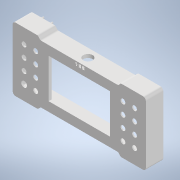
# Autodesk Inventor part: CONTROL_BOARD
Saved by Autodesk Inventor 2020 (Build 240168000, 168)
## iProperties
Created: 2020-06-05
Part Number: CONTROL_BOARD
Material: Generic
Document SubType Name: Modeling
Designer: Gebruiker
Density: 1 g/cm^3
Appearance: Default
Author: Gebruiker
Autodesk Inventor part; units mm, degrees
ref_plane "YZ Plane" through (0, 0, 0) normal (1, 0, 0) x (0, 1, 0)
ref_plane "XZ Plane" through (0, 0, 0) normal (0, 1, 0) x (-1, 0, 0)
ref_plane "XY Plane" through (0, 0, 0) normal (0, 0, 1) x (1, 0, 0)
sketch "Sketch1" plane through (0, 0, 0) normal (0, 0, 1) x (1, 0, 0)
  line L0 (-92.5, -50) -> (92.5, -50)
  line L1 (92.5, -50) -> (92.5, 50)
  line L2 (92.5, 50) -> (-92.5, 50)
  line L3 (-92.5, 50) -> (-92.5, -50)
  line L4 (-92.5, -50) -> (92.5, 50) construction
  line L5 (92.5, -50) -> (-92.5, 50) construction
  line L6 (70, 55) -> (115, 55)
  line L7 (115, 55) -> (115, 45)
  line L8 (115, 45) -> (70, 45)
  line L9 (70, 45) -> (70, 55)
  line L10 (70, 55) -> (115, 45) construction
  line L11 (115, 55) -> (70, 45) construction
  line L12 (70, -45) -> (115, -45)
  line L13 (115, -45) -> (115, -55)
  line L14 (115, -55) -> (70, -55)
  line L15 (70, -55) -> (70, -45)
  line L16 (70, -45) -> (115, -55) construction
  line L17 (115, -45) -> (70, -55) construction
  line L18 (-115, -45) -> (-70, -45)
  line L19 (-70, -45) -> (-70, -55)
  line L20 (-70, -55) -> (-115, -55)
  line L21 (-115, -55) -> (-115, -45)
  line L22 (-115, -45) -> (-70, -55) construction
  line L23 (-70, -45) -> (-115, -55) construction
  line L24 (-115, 55) -> (-70, 55)
  line L25 (-70, 55) -> (-70, 45)
  line L26 (-70, 45) -> (-115, 45)
  line L27 (-115, 45) -> (-115, 55)
  line L28 (-115, 55) -> (-70, 45) construction
  line L29 (-70, 55) -> (-115, 45) construction
  line L30 (70, 45) -> (115, 45)
  line L31 (115, 45) -> (115, -45)
  line L32 (115, -45) -> (70, -45)
  line L33 (70, -45) -> (70, 45)
  line L34 (70, 45) -> (115, -45) construction
  line L35 (115, 45) -> (70, -45) construction
  line L36 (-115, 45) -> (-70, 45)
  line L37 (-70, 45) -> (-70, -45)
  line L38 (-70, -45) -> (-115, -45)
  line L39 (-115, -45) -> (-115, 45)
  line L40 (-115, 45) -> (-70, -45) construction
  line L41 (-70, 45) -> (-115, -45) construction
  line L42 (115, 45) -> (115, 25)
  line L43 (115, -45) -> (115, -25)
  line L44 (-115, -45) -> (-115, -25)
  line L45 (-115, 45) -> (-115, 25)
  point P0 (0, 0)
  point P1 (92.5, 0)
  point P2 (-92.5, 0)
  point P3 (70, 50)
  point P4 (-70, 50)
  point P5 (-70, -50)
  point P6 (70, -50)
  dimension "d0" = 185
  dimension "d1" = 100
  dimension "d2" = 45
  dimension "d3" = 10
  dimension "d4" = 45
  dimension "d5" = 10
  dimension "d6" = 45
  dimension "d7" = 45
  dimension "d8" = 10
  dimension "d9" = 45
  dimension "d10" = 90
  dimension "d20" = 20
  dimension "d21" = 20
  dimension "d22" = 20
  dimension "d23" = 20
  dimension "d83" = 45
  constraints: 92 end point, 16 midpoint, 14 parallel, 7 horizontal, 7 perpendicular, 6 point on line, 1 collinear
  measures "d0" distance of L2.end L1.end
  measures "d1" distance of L1.end L0.end
  measures "d2" distance of L7.end L8.end
  measures "d3" distance of L6.end L7.end
  measures "d4" distance of L13.end L14.end
  measures "d5" distance of L12.end L13.end
  measures "d6" distance of L19.end L20.end
  measures "d7" distance of L25.end L26.end
  measures "d8" distance of L24.end L25.end
  measures "d9" distance of L31.end L32.end
  measures "d10" distance of L36.end L37.end
  measures "d20" distance of L7.end L42.end
  measures "d21" distance of L12.end L43.end
  measures "d22" distance of L18.start L44.end
  measures "d23" distance of L26.end L45.end
  measures "d83" distance of L37.end L38.end
extrude "Extrusion1" add sketch "Sketch1" against normal blind 30
fillet "Fillet1" radius 5 12 edges at (-115, 55, -15) (-115, -55, -15) (-70, -55, -15) (-70, -50, -15) (70, -50, -15) (70, -55, -15) (115, -55, -15) (115, 55, -15) (70, 55, -15) (70, 50, -15) (-70, 50, -15) (-70, 55, -15)
sketch "Sketch3" plane through (0, 0, 0) normal (0, 0, 1) x (1, 0, 0)
  line L0 (-5.942, 46.9465) -> (-3.942, 46.9465)
  line L1 (-3.942, 46.9465) -> (-3.942, 42.9465)
  line L2 (-3.942, 42.9465) -> (-5.942, 42.9465)
  line L3 (-5.942, 42.9465) -> (-5.942, 46.9465)
  line L4 (-5.942, 46.9465) -> (-3.942, 42.9465) construction
  line L5 (-3.942, 46.9465) -> (-5.942, 42.9465) construction
  line L6 (-6.942, 47.9465) -> (-2.942, 47.9465)
  line L7 (-2.942, 47.9465) -> (-2.942, 45.9465)
  line L8 (-2.942, 45.9465) -> (-6.942, 45.9465)
  line L9 (-6.942, 45.9465) -> (-6.942, 47.9465)
  line L10 (-6.942, 47.9465) -> (-2.942, 45.9465) construction
  line L11 (-2.942, 47.9465) -> (-6.942, 45.9465) construction
  line L12 (-1.0169, 47.9465) -> (2.9831, 47.9465)
  line L13 (2.9831, 47.9465) -> (2.9831, 46.4465)
  line L14 (2.9831, 46.4465) -> (-1.0169, 46.4465)
  line L15 (-1.0169, 46.4465) -> (-1.0169, 47.9465)
  line L16 (-1.0169, 46.1965) -> (2.9831, 46.1965)
  line L17 (2.9831, 46.1965) -> (2.9831, 44.6965)
  line L18 (2.9831, 44.6965) -> (-1.0169, 44.6965)
  line L19 (-1.0169, 44.6965) -> (-1.0169, 46.1965)
  line L20 (-1.0169, 42.9465) -> (2.9831, 42.9465)
  line L21 (2.9831, 42.9465) -> (2.9831, 44.4465)
  line L22 (2.9831, 44.4465) -> (-1.0169, 44.4465)
  line L23 (-1.0169, 44.4465) -> (-1.0169, 42.9465)
  line L24 (4.5797, 47.9465) -> (8.5797, 47.9465)
  line L25 (8.5797, 47.9465) -> (8.5797, 46.4465)
  line L26 (8.5797, 46.4465) -> (4.5797, 46.4465)
  line L27 (4.5797, 46.4465) -> (4.5797, 47.9465)
  line L28 (4.5797, 46.1965) -> (8.5797, 46.1965)
  line L29 (8.5797, 46.1965) -> (8.5797, 44.6965)
  line L30 (8.5797, 44.6965) -> (4.5797, 44.6965)
  line L31 (4.5797, 44.6965) -> (4.5797, 46.1965)
  line L32 (4.5797, 44.4465) -> (8.5797, 44.4465)
  line L33 (8.5797, 44.4465) -> (8.5797, 42.9465)
  line L34 (8.5797, 42.9465) -> (4.5797, 42.9465)
  line L35 (4.5797, 42.9465) -> (4.5797, 44.4465)
  point P0 (0, 0)
  point P1 (-4.942, 44.9465)
  point P2 (-4.942, 46.9465)
  point P3 (-5.942, 45.9465)
  point P4 (-3.942, 45.9465)
  dimension "d26" = 2
  dimension "d27" = 4
  dimension "d28" = 4
  dimension "d29" = 2
  dimension "d30" = 4
  dimension "d31" = 1.5
  dimension "d32" = 4
  dimension "d33" = 1.5
  dimension "d34" = 4
  dimension "d35" = 1.5
  dimension "d36" = 0.25
  dimension "d37" = 0.25
  dimension "d38" = 4
  dimension "d39" = 1.5
  dimension "d40" = 4
  dimension "d41" = 1.5
  dimension "d42" = 4
  constraints: 72 end point, 16 parallel, 8 horizontal, 8 perpendicular, 5 midpoint, 3 point on line
  measures "d26" distance of L1.end L2.end
  measures "d27" distance of L0.end L1.end
  measures "d28" distance of L7.end L8.end
  measures "d29" distance of L6.end L7.end
  measures "d30" distance of L13.end L14.end
  measures "d31" distance of L12.end L13.end
  measures "d32" distance of L17.end L18.end
  measures "d33" distance of L16.end L17.end
  measures "d34" distance of L22.end L21.end
  measures "d35" distance of L21.end L20.end
  measures "d36" distance between parallel lines of L16 L14
  measures "d37" distance between parallel lines of L22 L18
  measures "d38" distance of L25.end L26.end
  measures "d39" distance of L24.end L25.end
  measures "d40" distance of L29.end L30.end
  measures "d41" distance of L28.end L29.end
  measures "d42" distance of L33.end L34.end
extrude "Extrusion3" cut sketch "Sketch3" against normal blind 2
sketch "Sketch5" plane through (0, 0, -30) normal (0, 0, -1) x (-1, 0, 0)
  line L0 (-109, 44) -> (109, 44)
  line L1 (109, 44) -> (109, -44)
  line L2 (109, -44) -> (-109, -44)
  line L3 (-109, -44) -> (-109, 44)
  line L4 (-109, 44) -> (109, -44) construction
  line L5 (109, 44) -> (-109, -44) construction
  point P0 (0, 0)
  dimension "d51" = 218
  dimension "d52" = 88
  constraints: 12 end point, 2 midpoint, 2 parallel, 1 horizontal, 1 perpendicular
  measures "d51" distance of L1.end L2.end
  measures "d52" distance of L0.end L1.end
extrude "Extrusion5" cut sketch "Sketch5" against normal blind 25
sketch "Sketch6" plane through (0, 0, 0) normal (0, 0, 1) x (1, 0, 0)
  line L0 (-53, 34) -> (53, 34)
  line L1 (53, 34) -> (53, -34)
  line L2 (53, -34) -> (-53, -34)
  line L3 (-53, -34) -> (-53, 34)
  line L4 (-53, 34) -> (53, -34) construction
  line L5 (53, 34) -> (-53, -34) construction
  point P0 (0, 0)
  dimension "d56" = 106
  dimension "d57" = 68
  constraints: 12 end point, 2 midpoint, 2 parallel, 1 horizontal, 1 perpendicular
  measures "d56" distance of L1.end L2.end
  measures "d57" distance of L0.end L1.end
extrude "Extrusion6" cut sketch "Sketch6" against normal blind 5
sketch "Sketch7" plane through (0, 0, 0) normal (0, 0, 1) x (1, 0, 0)
  line L0 (-53, -34) -> (-53, 34) projected
  line L1 (-53, 34) -> (53, 34) projected
  line L2 (53, 34) -> (53, -34) projected
  line L3 (53, -34) -> (-53, -34) projected
  line L4 (2.9831, 44.6965) -> (-1.0169, 44.6965) projected
  line L5 (-1.0169, 44.6965) -> (-1.0169, 46.1965) projected
  line L6 (-1.0169, 46.1965) -> (2.9831, 46.1965) projected
  line L7 (2.9831, 46.1965) -> (2.9831, 44.6965) projected
  line L8 (8.5797, 46.4465) -> (4.5797, 46.4465) projected
  line L9 (4.5797, 46.4465) -> (4.5797, 47.9465) projected
  line L10 (4.5797, 47.9465) -> (8.5797, 47.9465) projected
  line L11 (8.5797, 47.9465) -> (8.5797, 46.4465) projected
  line L12 (-1.0169, 44.4465) -> (2.9831, 44.4465) projected
  line L13 (2.9831, 44.4465) -> (2.9831, 42.9465) projected
  line L14 (2.9831, 42.9465) -> (-1.0169, 42.9465) projected
  line L15 (-1.0169, 42.9465) -> (-1.0169, 44.4465) projected
  line L16 (-1.0169, 46.4465) -> (-1.0169, 47.9465) projected
  line L17 (-1.0169, 47.9465) -> (2.9831, 47.9465) projected
  line L18 (2.9831, 47.9465) -> (2.9831, 46.4465) projected
  line L19 (2.9831, 46.4465) -> (-1.0169, 46.4465) projected
  line L20 (4.5797, 46.1965) -> (8.5797, 46.1965) projected
  line L21 (8.5797, 46.1965) -> (8.5797, 44.6965) projected
  line L22 (8.5797, 44.6965) -> (4.5797, 44.6965) projected
  line L23 (4.5797, 44.6965) -> (4.5797, 46.1965) projected
  line L24 (4.5797, 42.9465) -> (4.5797, 44.4465) projected
  line L25 (4.5797, 44.4465) -> (8.5797, 44.4465) projected
  line L26 (8.5797, 44.4465) -> (8.5797, 42.9465) projected
  line L27 (8.5797, 42.9465) -> (4.5797, 42.9465) projected
  line L28 (-3.942, 45.9465) -> (-3.942, 42.9465) projected
  line L29 (-3.942, 42.9465) -> (-5.942, 42.9465) projected
  line L30 (-5.942, 42.9465) -> (-5.942, 45.9465) projected
  line L31 (-5.942, 45.9465) -> (-6.942, 45.9465) projected
  line L32 (-6.942, 45.9465) -> (-6.942, 47.9465) projected
  line L33 (-6.942, 47.9465) -> (-2.942, 47.9465) projected
  line L34 (-2.942, 47.9465) -> (-2.942, 45.9465) projected
  line L35 (-2.942, 45.9465) -> (-3.942, 45.9465) projected
  arc A0 (-69.3301, 52.5) -> (-73.6603, 55) centre (-73.6603, 50) ccw projected
  line L36 (-73.6603, 55) -> (-110, 55) projected
  arc A1 (-110, 55) -> (-115, 50) centre (-110, 50) ccw projected
  arc A2 (-115, -50) -> (-110, -55) centre (-110, -50) ccw projected
  line L37 (-110, -55) -> (-73.6603, -55) projected
  arc A3 (-73.6603, -55) -> (-69.3301, -52.5) centre (-73.6603, -50) ccw projected
  arc A4 (-65, -50) -> (-69.3301, -52.5) centre (-65, -55) ccw projected
  line L38 (-65, -50) -> (65, -50) projected
  arc A5 (69.3301, -52.5) -> (65, -50) centre (65, -55) ccw projected
  arc A6 (69.3301, -52.5) -> (73.6603, -55) centre (73.6603, -50) ccw projected
  line L39 (73.6603, -55) -> (110, -55) projected
  arc A7 (110, -55) -> (115, -50) centre (110, -50) ccw projected
  arc A8 (115, 50) -> (110, 55) centre (110, 50) ccw projected
  line L40 (110, 55) -> (73.6603, 55) projected
  arc A9 (73.6603, 55) -> (69.3301, 52.5) centre (73.6603, 50) ccw projected
  arc A10 (65, 50) -> (69.3301, 52.5) centre (65, 55) ccw projected
  line L41 (65, 50) -> (-65, 50) projected
  arc A11 (-69.3301, 52.5) -> (-65, 50) centre (-65, 55) ccw projected
  line L42 (4.825, 59.0166) -> (4.825, -53.5355) construction
  line L43 (-115, 50) -> (-115, -50) projected
  line L44 (115, -50) -> (115, 50) projected
  point P0 (0, 0)
  constraints: 2 end point, 1 vertical
sketch "Sketch8" plane through (0, 0, 0) normal (0, 0, 1) x (1, 0, 0)
  line L0 (67.7, 35.96) -> (83, 35.96)
  line L1 (83, 35.96) -> (83, 23.66)
  line L2 (83, 23.66) -> (67.7, 23.66)
  line L3 (67.7, 23.66) -> (67.7, 35.96)
  line L4 (87.7, 35.96) -> (103, 35.96)
  line L5 (103, 35.96) -> (103, 23.66)
  line L6 (103, 23.66) -> (87.7, 23.66)
  line L7 (87.7, 23.66) -> (87.7, 35.96)
  line L8 (67.7, 16.08) -> (83, 16.08)
  line L9 (83, 16.08) -> (83, 3.78)
  line L10 (83, 3.78) -> (67.7, 3.78)
  line L11 (67.7, 3.78) -> (67.7, 16.08)
  line L12 (87.7, 16.08) -> (103, 16.08)
  line L13 (103, 16.08) -> (103, 3.78)
  line L14 (103, 3.78) -> (87.7, 3.78)
  line L15 (87.7, 3.78) -> (87.7, 16.08)
  line L16 (-123.4592, 0) -> (132.261, 0) construction
  line L17 (0, 57.3995) -> (0, -58.2893) construction
  line L18 (67.7, -35.96) -> (83, -35.96)
  line L19 (83, -35.96) -> (83, -23.66)
  line L20 (83, -23.66) -> (67.7, -23.66)
  line L21 (67.7, -23.66) -> (67.7, -35.96)
  line L22 (87.7, -35.96) -> (103, -35.96)
  line L23 (103, -35.96) -> (103, -23.66)
  line L24 (103, -23.66) -> (87.7, -23.66)
  line L25 (87.7, -23.66) -> (87.7, -35.96)
  line L26 (67.7, -16.08) -> (83, -16.08)
  line L27 (83, -16.08) -> (83, -3.78)
  line L28 (83, -3.78) -> (67.7, -3.78)
  line L29 (67.7, -3.78) -> (67.7, -16.08)
  line L30 (87.7, -16.08) -> (103, -16.08)
  line L31 (103, -16.08) -> (103, -3.78)
  line L32 (103, -3.78) -> (87.7, -3.78)
  line L33 (87.7, -3.78) -> (87.7, -16.08)
  line L34 (-67.7, 35.96) -> (-83, 35.96)
  line L35 (-83, 35.96) -> (-83, 23.66)
  line L36 (-83, 23.66) -> (-67.7, 23.66)
  line L37 (-67.7, 23.66) -> (-67.7, 35.96)
  line L38 (-87.7, 35.96) -> (-103, 35.96)
  line L39 (-103, 35.96) -> (-103, 23.66)
  line L40 (-103, 23.66) -> (-87.7, 23.66)
  line L41 (-87.7, 23.66) -> (-87.7, 35.96)
  line L42 (-67.7, 16.08) -> (-83, 16.08)
  line L43 (-83, 16.08) -> (-83, 3.78)
  line L44 (-83, 3.78) -> (-67.7, 3.78)
  line L45 (-67.7, 3.78) -> (-67.7, 16.08)
  line L46 (-87.7, 16.08) -> (-103, 16.08)
  line L47 (-103, 16.08) -> (-103, 3.78)
  line L48 (-103, 3.78) -> (-87.7, 3.78)
  line L49 (-87.7, 3.78) -> (-87.7, 16.08)
  line L50 (-67.7, -35.96) -> (-83, -35.96)
  line L51 (-67.7, -23.66) -> (-67.7, -35.96)
  line L52 (-83, -23.66) -> (-67.7, -23.66)
  line L53 (-83, -35.96) -> (-83, -23.66)
  line L54 (-87.7, -23.66) -> (-87.7, -35.96)
  line L55 (-103, -23.66) -> (-87.7, -23.66)
  line L56 (-103, -35.96) -> (-103, -23.66)
  line L57 (-87.7, -35.96) -> (-103, -35.96)
  line L58 (-67.7, -16.08) -> (-83, -16.08)
  line L59 (-67.7, -3.78) -> (-67.7, -16.08)
  line L60 (-83, -3.78) -> (-67.7, -3.78)
  line L61 (-83, -16.08) -> (-83, -3.78)
  line L62 (-87.7, -3.78) -> (-87.7, -16.08)
  line L63 (-87.7, -16.08) -> (-103, -16.08)
  line L64 (-103, -16.08) -> (-103, -3.78)
  line L65 (-103, -3.78) -> (-87.7, -3.78)
  line L66 (-174.6033, 0) -> (183.4051, 0) projected
  line L67 (115, -50) -> (115, 50) projected
  line L68 (-115, 50) -> (-115, -50) projected
  line L69 (75.35, 35.96) -> (75.35, 23.66) construction
  line L70 (95.35, 35.96) -> (95.35, 23.66) construction
  point P0 (0, 0)
  dimension "d106" = 15.3
  dimension "d107" = 12.3
  dimension "d108" = 15.3
  dimension "d109" = 12.3
  dimension "d110" = 7.58
  dimension "d112" = 3.78
  dimension "d113" = 12
  dimension "d115" = 12
  dimension "d128" = 20
  dimension "d150" = 7.58
  constraints: 136 end point, 48 symmetric about line, 32 point on line, 8 parallel, 5 horizontal, 4 midpoint, 4 perpendicular, 1 collinear, 1 vertical
  measures "d106" distance of L1.end L2.end
  measures "d107" distance of L0.end L1.end
  measures "d108" distance of L5.end L6.end
  measures "d109" distance of L8.end L9.end
  measures "d110" distance between parallel lines of L12 L6
  measures "d112" distance between parallel lines of L16 L14
  measures "d113" distance between parallel lines of L67 L5
  measures "d115" distance between parallel lines of L68 L39
  measures "d128" distance between parallel lines of L70 L69
  measures "d150" distance between parallel lines of L24 L30
extrude "Extrusion10" cut sketch "Sketch8" against normal blind 5
sketch "Sketch9" plane through (0, 0, 0) normal (0, 0, 1) x (1, 0, 0)
  line L0 (109, 44) -> (-109, 44) projected
  line L1 (83, 3.78) -> (67.7, 3.78) projected
  line L2 (67.7, 3.78) -> (67.7, 16.08) projected
  line L3 (67.7, 16.08) -> (83, 16.08) projected
  line L4 (83, 16.08) -> (83, 3.78) projected
  line L5 (83, -35.96) -> (67.7, -35.96) projected
  line L6 (67.7, -35.96) -> (67.7, -23.66) projected
  line L7 (67.7, -23.66) -> (83, -23.66) projected
  line L8 (83, -23.66) -> (83, -35.96) projected
  line L9 (-67.7, 16.08) -> (-67.7, 3.78) projected
  line L10 (-67.7, 3.78) -> (-83, 3.78) projected
  line L11 (-83, 3.78) -> (-83, 16.08) projected
  line L12 (-83, 16.08) -> (-67.7, 16.08) projected
  line L13 (-87.7, -35.96) -> (-103, -35.96) projected
  line L14 (-103, -35.96) -> (-103, -23.66) projected
  line L15 (-103, -23.66) -> (-87.7, -23.66) projected
  line L16 (-87.7, -23.66) -> (-87.7, -35.96) projected
  line L17 (-87.7, -3.78) -> (-87.7, -16.08) projected
  line L18 (-87.7, -16.08) -> (-103, -16.08) projected
  line L19 (-103, -16.08) -> (-103, -3.78) projected
  line L20 (-103, -3.78) -> (-87.7, -3.78) projected
  line L21 (-87.7, 35.96) -> (-87.7, 23.66) projected
  line L22 (-87.7, 23.66) -> (-103, 23.66) projected
  line L23 (-103, 23.66) -> (-103, 35.96) projected
  line L24 (-103, 35.96) -> (-87.7, 35.96) projected
  line L25 (103, -16.08) -> (87.7, -16.08) projected
  line L26 (87.7, -16.08) -> (87.7, -3.78) projected
  line L27 (87.7, -3.78) -> (103, -3.78) projected
  line L28 (103, -3.78) -> (103, -16.08) projected
  line L29 (103, 35.96) -> (103, 23.66) projected
  line L30 (103, 23.66) -> (87.7, 23.66) projected
  line L31 (87.7, 23.66) -> (87.7, 35.96) projected
  line L32 (87.7, 35.96) -> (103, 35.96) projected
  line L33 (87.7, 3.78) -> (87.7, 16.08) projected
  line L34 (87.7, 16.08) -> (103, 16.08) projected
  line L35 (103, 16.08) -> (103, 3.78) projected
  line L36 (103, 3.78) -> (87.7, 3.78) projected
  line L37 (103, -35.96) -> (87.7, -35.96) projected
  line L38 (87.7, -35.96) -> (87.7, -23.66) projected
  line L39 (87.7, -23.66) -> (103, -23.66) projected
  line L40 (103, -23.66) -> (103, -35.96) projected
  line L41 (-87.7, 16.08) -> (-87.7, 3.78) projected
  line L42 (-87.7, 3.78) -> (-103, 3.78) projected
  line L43 (-103, 3.78) -> (-103, 16.08) projected
  line L44 (-103, 16.08) -> (-87.7, 16.08) projected
  line L45 (-83, -35.96) -> (-83, -23.66) projected
  line L46 (-83, -23.66) -> (-67.7, -23.66) projected
  line L47 (-67.7, -23.66) -> (-67.7, -35.96) projected
  line L48 (-67.7, -35.96) -> (-83, -35.96) projected
  line L49 (-83, -3.78) -> (-67.7, -3.78) projected
  line L50 (-67.7, -3.78) -> (-67.7, -16.08) projected
  line L51 (-67.7, -16.08) -> (-83, -16.08) projected
  line L52 (-83, -16.08) -> (-83, -3.78) projected
  line L53 (-83, 35.96) -> (-67.7, 35.96) projected
  line L54 (-67.7, 35.96) -> (-67.7, 23.66) projected
  line L55 (-67.7, 23.66) -> (-83, 23.66) projected
  line L56 (-83, 23.66) -> (-83, 35.96) projected
  line L57 (67.7, -3.78) -> (83, -3.78) projected
  line L58 (83, -3.78) -> (83, -16.08) projected
  line L59 (83, -16.08) -> (67.7, -16.08) projected
  line L60 (67.7, -16.08) -> (67.7, -3.78) projected
  line L61 (83, 35.96) -> (83, 23.66) projected
  line L62 (83, 23.66) -> (67.7, 23.66) projected
  line L63 (67.7, 23.66) -> (67.7, 35.96) projected
  line L64 (67.7, 35.96) -> (83, 35.96) projected
  line L65 (-53, 34) -> (53, 34) projected
  line L66 (53, 34) -> (53, -34) projected
  line L67 (53, -34) -> (-53, -34) projected
  line L68 (-53, -34) -> (-53, 34) projected
  line L69 (2.9831, 44.6965) -> (-1.0169, 44.6965) projected
  line L70 (-1.0169, 44.6965) -> (-1.0169, 46.1965) projected
  line L71 (-1.0169, 46.1965) -> (2.9831, 46.1965) projected
  line L72 (2.9831, 46.1965) -> (2.9831, 44.6965) projected
  line L73 (4.5797, 46.4465) -> (4.5797, 47.9465) projected
  line L74 (4.5797, 47.9465) -> (8.5797, 47.9465) projected
  line L75 (8.5797, 47.9465) -> (8.5797, 46.4465) projected
  line L76 (8.5797, 46.4465) -> (4.5797, 46.4465) projected
  line L77 (2.9831, 44.4465) -> (2.9831, 42.9465) projected
  line L78 (2.9831, 42.9465) -> (-1.0169, 42.9465) projected
  line L79 (-1.0169, 42.9465) -> (-1.0169, 44.4465) projected
  line L80 (-1.0169, 44.4465) -> (2.9831, 44.4465) projected
  line L81 (-1.0169, 46.4465) -> (-1.0169, 47.9465) projected
  line L82 (-1.0169, 47.9465) -> (2.9831, 47.9465) projected
  line L83 (2.9831, 47.9465) -> (2.9831, 46.4465) projected
  line L84 (2.9831, 46.4465) -> (-1.0169, 46.4465) projected
  line L85 (4.5797, 46.1965) -> (8.5797, 46.1965) projected
  line L86 (8.5797, 46.1965) -> (8.5797, 44.6965) projected
  line L87 (8.5797, 44.6965) -> (4.5797, 44.6965) projected
  line L88 (4.5797, 44.6965) -> (4.5797, 46.1965) projected
  line L89 (4.5797, 44.4465) -> (8.5797, 44.4465) projected
  line L90 (8.5797, 44.4465) -> (8.5797, 42.9465) projected
  line L91 (8.5797, 42.9465) -> (4.5797, 42.9465) projected
  line L92 (4.5797, 42.9465) -> (4.5797, 44.4465) projected
  line L93 (-2.942, 47.9465) -> (-2.942, 45.9465) projected
  line L94 (-2.942, 45.9465) -> (-3.942, 45.9465) projected
  line L95 (-3.942, 45.9465) -> (-3.942, 42.9465) projected
  line L96 (-3.942, 42.9465) -> (-5.942, 42.9465) projected
  line L97 (-5.942, 42.9465) -> (-5.942, 45.9465) projected
  line L98 (-5.942, 45.9465) -> (-6.942, 45.9465) projected
  line L99 (-6.942, 45.9465) -> (-6.942, 47.9465) projected
  line L100 (-6.942, 47.9465) -> (-2.942, 47.9465) projected
  arc A0 (-69.3301, 52.5) -> (-73.6603, 55) centre (-73.6603, 50) ccw projected
  line L101 (-73.6603, 55) -> (-110, 55) projected
  arc A1 (-110, 55) -> (-115, 50) centre (-110, 50) ccw projected
  line L102 (-115, 50) -> (-115, -50) projected
  arc A2 (-115, -50) -> (-110, -55) centre (-110, -50) ccw projected
  line L103 (-110, -55) -> (-73.6603, -55) projected
  arc A3 (-73.6603, -55) -> (-69.3301, -52.5) centre (-73.6603, -50) ccw projected
  arc A4 (-65, -50) -> (-69.3301, -52.5) centre (-65, -55) ccw projected
  line L104 (-65, -50) -> (65, -50) projected
  arc A5 (69.3301, -52.5) -> (65, -50) centre (65, -55) ccw projected
  arc A6 (69.3301, -52.5) -> (73.6603, -55) centre (73.6603, -50) ccw projected
  line L105 (73.6603, -55) -> (110, -55) projected
  arc A7 (110, -55) -> (115, -50) centre (110, -50) ccw projected
  line L106 (115, -50) -> (115, 50) projected
  arc A8 (115, 50) -> (110, 55) centre (110, 50) ccw projected
  line L107 (110, 55) -> (73.6603, 55) projected
  arc A9 (73.6603, 55) -> (69.3301, 52.5) centre (73.6603, 50) ccw projected
  arc A10 (65, 50) -> (69.3301, 52.5) centre (65, 55) ccw projected
  line L108 (65, 50) -> (-65, 50) projected
  arc A11 (-69.3301, 52.5) -> (-65, 50) centre (-65, 55) ccw projected
  circle A12 centre (-95.35, 29.81) radius 4.15
  circle A13 centre (-75.35, 29.81) radius 4.15
  circle A14 centre (-95.35, 9.93) radius 4.15
  circle A15 centre (-75.35, 9.93) radius 4.15
  line L109 (-132.2641, 0) -> (122.8696, 0) construction
  line L110 (0, 58.5918) -> (0, -75.697) construction
  circle A16 centre (-95.35, -29.81) radius 4.15
  circle A17 centre (-75.35, -29.81) radius 4.15
  circle A18 centre (-95.35, -9.93) radius 4.15
  circle A19 centre (-75.35, -9.93) radius 4.15
  circle A20 centre (95.35, 29.81) radius 4.15
  circle A21 centre (75.35, 29.81) radius 4.15
  circle A22 centre (95.35, 9.93) radius 4.15
  circle A23 centre (75.35, 9.93) radius 4.15
  circle A24 centre (95.35, -29.81) radius 4.15
  circle A25 centre (75.35, -29.81) radius 4.15
  circle A26 centre (75.35, -9.93) radius 4.15
  circle A27 centre (95.35, -9.93) radius 4.15
  line L111 (-103, 16.08) -> (-87.7, 16.08) projected
  line L112 (-1.0169, 46.9465) -> (0, 46.9465)
  line L113 (0, 46.9465) -> (0, 45.9465)
  line L114 (0, 45.9465) -> (-1.0169, 45.9465)
  line L115 (-1.0169, 45.9465) -> (-1.0169, 46.9465)
  line L116 (8.5797, 44.6965) -> (4.5797, 44.6965) projected
  line L117 (109, 44) -> (-109, 44) projected
  line L118 (8.5797, 44.6965) -> (7.5636, 44.6965)
  line L119 (7.5636, 44.6965) -> (7.5636, 44)
  line L120 (7.5636, 44) -> (8.5797, 44)
  line L121 (8.5797, 44) -> (8.5797, 44.6965)
  point P0 (0, 0)
  point P1 (-75.35, 35.96)
  point P2 (-95.35, 35.96)
  point P3 (-95.35, 16.08)
  point P4 (-95.35, 16.08)
  point P5 (-95.35, 16.08)
  point P6 (-75.35, 16.08)
  point P7 (-75.35, -3.78)
  point P8 (-95.35, -3.78)
  point P9 (-95.35, -23.66)
  point P10 (-75.35, -23.66)
  point P11 (-67.7, -9.93)
  point P12 (95.35, 35.96)
  point P13 (7.5636, 44.4465)
  point P14 (0, 46.1965)
  point P15 (0, 46.4465)
  dimension "d118" = 8.3
  dimension "d119" = 8.3
  dimension "d120" = 8.3
  dimension "d121" = 8.3
  dimension "d126" = 20
  dimension "d129" = 20
  dimension "d130" = 6.15
  dimension "d131" = 6.15
  constraints: 20 end point, 16 centre point, 12 midpoint, 12 symmetric about line, 11 vertical alignment, 4 parallel, 3 horizontal, 3 point on line, 2 perpendicular, 1 horizontal alignment, 1 vertical, 12 other
  measures "d118" diameter of A12
  measures "d119" diameter of A13
  measures "d120" diameter of A14
  measures "d121" diameter of A15
  measures "d126" distance of A13.centre A12.centre
  measures "d129" distance of A15.centre A14.centre
  measures "d130" distance from line of A13.centre L53
  measures "d131" distance from line of A15.centre L12
extrude "Extrusion11" cut sketch "Sketch9" against normal blind 2 contours L89 L119 L87 L121 | L1 L2 L3 L4 | L5 L6 L7 L8 | L9 L10 L11 L12 | L13 L14 L15 L16 | L17 L18 L19 L20 | L21 L22 L23 L24 | L25 L26 L27 L28 | L29 L30 L31 L32 | L33 L34 L35 L36 | L37 L38 L39 L40 | L41 L42 L43 L44 | L45 L46 L47 L48 | L49 L50 L51 L52 | L53 L54 L55 L56 | L57 L58 L59 L60 | L61 L62 L63 L64 | L71 L115 L84 L113 | A17
extrude "Extrusion12" add sketch "Sketch9" against normal blind 2 contours L1 L2 L3 L4 | L5 L6 L7 L8 | L9 L10 L11 L12 | L13 L14 L15 L16 | L17 L18 L19 L20 | L21 L22 L23 L24 | L25 L26 L27 L28 | L29 L30 L31 L32 | L33 L34 L35 L36 | L37 L38 L39 L40 | L41 L42 L43 L44 | L45 L46 L47 L48 | L49 L50 L51 L52 | L53 L54 L55 L56 | L57 L58 L59 L60 | L61 L62 L63 L64 | A11 L108 A10 A9 L107 A8 L106 A7 L105 A6 A5 L104 A4 A3 L103 A2 L102 A1 L101 A0
sketch "Sketch13" plane through (0, 0, -30) normal (0, 0, -1) x (-1, 0, 0)
  line L0 (-109, 44) -> (109, 44) projected
  line L1 (101, 44) -> (80.8, 44)
  line L2 (80.8, 44) -> (80.8, 52.2)
  line L3 (80.8, 52.2) -> (101, 52.2)
  line L4 (101, 52.2) -> (101, 44)
  line L5 (115, -50) -> (115, 50) projected
  point P0 (0, 0)
  dimension "d151" = 20.2
  dimension "d152" = 8.2
  dimension "d153" = 14
  constraints: 8 end point, 2 parallel, 1 horizontal, 1 perpendicular, 1 point on line
  measures "d151" distance of L2.end L3.end
  measures "d152" distance of L1.end L2.end
  measures "d153" distance between parallel lines of L5 L4
extrude "Extrusion16" cut sketch "Sketch13" against normal blind 2.2
mirror "Mirror3" about plane through (0, 0, 0) normal (1, 0, 0) of "Extrusion16"
sketch "Sketch14" plane through (-65, 50, -30) normal (0, 1, 0) x (1, 0, 0)
  circle A0 centre (65, -15) radius 8
  line L0 (0, 0) -> (130, 0) projected
  line L1 (65, -15) -> (65, 0) construction
  line L2 (130, 0) -> (0, 0) construction
  line L3 (65, -30) -> (65, -15) construction
  line L4 (12, -25) -> (118, -25) construction
  dimension "d156" = 16
  constraints: 4 end point, 1 centre point, 1 collinear, 1 midpoint, 1 perpendicular
  measures "d156" diameter of A0
extrude "Extrusion17" cut sketch "Sketch14" against normal blind 7
sketch "Sketch15" plane through (0, 0, 0) normal (0, 0, 1) x (1, 0, 0)
  circle A0 centre (-95.35, -29.81) radius 4.15 projected
  circle A1 centre (-95.35, -29.81) radius 5
  point P0 (0, 0)
  dimension "d160" = 10
  constraints: 1 centre point, 1 coincident
  measures "d160" diameter of A1
extrude "Extrusion18" cut sketch "Sketch15" against normal blind 7
sketch "Sketch17" plane through (0, 0, -5) normal (0, 0, -1) x (-1, 0, 0)
  circle A0 centre (102.9761, 38.9853) radius 1.5 projected
  circle A1 centre (65.4761, 38.9853) radius 1.5 projected
  circle A2 centre (102.9761, -38.5147) radius 1.5 projected
  circle A3 centre (65.4761, -38.5147) radius 1.5 projected
  circle A4 centre (56.7761, -33.5647) radius 1.6 projected
  circle A5 centre (56.7761, 33.9353) radius 1.6 projected
  circle A6 centre (-56.7239, 33.9353) radius 1.6 projected
  circle A7 centre (-56.7239, -33.5647) radius 1.6 projected
  line L0 (-67.7, 16.08) -> (-67.7, 3.78) projected
  line L1 (-67.7, 3.78) -> (-83, 3.78) projected
  line L2 (-83, 3.78) -> (-83, 16.08) projected
  line L3 (-83, 16.08) -> (-67.7, 16.08) projected
  line L4 (-67.7, -23.66) -> (-67.7, -35.96) projected
  line L5 (-67.7, -35.96) -> (-83, -35.96) projected
  line L6 (-83, -35.96) -> (-83, -23.66) projected
  line L7 (-83, -23.66) -> (-67.7, -23.66) projected
  line L8 (83, 3.78) -> (67.7, 3.78) projected
  line L9 (67.7, 3.78) -> (67.7, 16.08) projected
  line L10 (67.7, 16.08) -> (83, 16.08) projected
  line L11 (83, 16.08) -> (83, 3.78) projected
  line L12 (103, -23.66) -> (103, -35.96) projected
  line L13 (103, -35.96) -> (87.7, -35.96) projected
  line L14 (87.7, -35.96) -> (87.7, -23.66) projected
  line L15 (87.7, -23.66) -> (103, -23.66) projected
  line L16 (103, -16.08) -> (87.7, -16.08) projected
  line L17 (87.7, -16.08) -> (87.7, -3.78) projected
  line L18 (87.7, -3.78) -> (103, -3.78) projected
  line L19 (103, -3.78) -> (103, -16.08) projected
  line L20 (103, 23.66) -> (87.7, 23.66) projected
  line L21 (87.7, 23.66) -> (87.7, 35.96) projected
  line L22 (87.7, 35.96) -> (103, 35.96) projected
  line L23 (103, 35.96) -> (103, 23.66) projected
  line L24 (-87.7, -3.78) -> (-87.7, -16.08) projected
  line L25 (-87.7, -16.08) -> (-103, -16.08) projected
  line L26 (-103, -16.08) -> (-103, -3.78) projected
  line L27 (-103, -3.78) -> (-87.7, -3.78) projected
  line L28 (-87.7, 23.66) -> (-103, 23.66) projected
  line L29 (-103, 23.66) -> (-103, 35.96) projected
  line L30 (-103, 35.96) -> (-87.7, 35.96) projected
  line L31 (-87.7, 35.96) -> (-87.7, 23.66) projected
  line L32 (-103, 16.08) -> (-87.7, 16.08) projected
  line L33 (-87.7, 16.08) -> (-87.7, 3.78) projected
  line L34 (-87.7, 3.78) -> (-103, 3.78) projected
  line L35 (-103, 3.78) -> (-103, 16.08) projected
  line L36 (-87.7, -23.66) -> (-87.7, -35.96) projected
  line L37 (-87.7, -35.96) -> (-103, -35.96) projected
  line L38 (-103, -35.96) -> (-103, -23.66) projected
  line L39 (-103, -23.66) -> (-87.7, -23.66) projected
  line L40 (103, 3.78) -> (87.7, 3.78) projected
  line L41 (87.7, 3.78) -> (87.7, 16.08) projected
  line L42 (87.7, 16.08) -> (103, 16.08) projected
  line L43 (103, 16.08) -> (103, 3.78) projected
  line L44 (67.7, -23.66) -> (83, -23.66) projected
  line L45 (83, -23.66) -> (83, -35.96) projected
  line L46 (83, -35.96) -> (67.7, -35.96) projected
  line L47 (67.7, -35.96) -> (67.7, -23.66) projected
  line L48 (67.7, -16.08) -> (67.7, -3.78) projected
  line L49 (67.7, -3.78) -> (83, -3.78) projected
  line L50 (83, -3.78) -> (83, -16.08) projected
  line L51 (83, -16.08) -> (67.7, -16.08) projected
  line L52 (67.7, 23.66) -> (67.7, 35.96) projected
  line L53 (67.7, 35.96) -> (83, 35.96) projected
  line L54 (83, 35.96) -> (83, 23.66) projected
  line L55 (83, 23.66) -> (67.7, 23.66) projected
  line L56 (-83, -16.08) -> (-83, -3.78) projected
  line L57 (-83, -3.78) -> (-67.7, -3.78) projected
  line L58 (-67.7, -3.78) -> (-67.7, -16.08) projected
  line L59 (-67.7, -16.08) -> (-83, -16.08) projected
  line L60 (-67.7, 23.66) -> (-83, 23.66) projected
  line L61 (-83, 23.66) -> (-83, 35.96) projected
  line L62 (-83, 35.96) -> (-67.7, 35.96) projected
  line L63 (-67.7, 35.96) -> (-67.7, 23.66) projected
  line L64 (-53, 34) -> (53, 34) projected
  line L65 (53, 34) -> (53, -34) projected
  line L66 (53, -34) -> (-53, -34) projected
  line L67 (-53, -34) -> (-53, 34) projected
  line L68 (-109, 44) -> (109, 44) projected
  line L69 (-109, -44) -> (-109, 44) projected
  line L70 (109, -44) -> (-109, -44) projected
  line L71 (109, 44) -> (109, -44) projected
  circle A8 centre (-65.4239, -38.5147) radius 1.5 projected
  circle A9 centre (-102.9239, -38.5147) radius 1.5 projected
  circle A10 centre (-102.9239, 38.9853) radius 1.5 projected
  circle A11 centre (-65.4239, 38.9853) radius 1.5 projected
  point P0 (0, 0)
hole "Hole1" at (-102.9761, 38.9853, -5) at (-102.9761, -38.5147, -5) at (-65.4761, -38.5147, -5) at (-56.7761, -33.5647, -5) at (-65.4761, 38.9853, -5) at (-56.7761, 33.9353, -5) at (56.7239, -33.5647, -5) at (56.7239, 33.9353, -5) at (65.4239, 38.9853, -5) at (102.9239, 38.9853, -5) at (102.9239, -38.5147, -5) at (65.4239, -38.5147, -5) direction (0, 0, 1) diameter 2.459 depth 2 tip angle 118 thread size "M3x0.5" class "6H" standard "ISO Metric profile"
body "Solid1"
